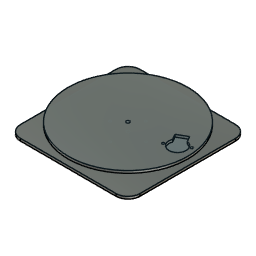
Bases v9 (Autodesk Fusion 360 design; units mm, degrees)
Autodesk Fusion 360 part; units mm, degrees
sketch "Sketch1" plane through (0, 0, 0) normal (0, 0, 1) x (1, 0, 0)
  line L0 (-100, 100) -> (100, 100)
  line L1 (100, 100) -> (100, -100)
  line L2 (100, -100) -> (-100, -100)
  line L3 (-100, -100) -> (-100, 100)
  circle A0 centre (0, 0) radius 65 construction
  circle A1 centre (30, 0) radius 2
  circle A2 centre (0, 30) radius 2
  circle A3 centre (-30, 0) radius 2
  circle A4 centre (0, -30) radius 2
  circle A5 centre (0, 0) radius 2.8
  point P0 (0, -100)
  point P1 (-100, 0)
  dimension "d1" = 200
  dimension "d2" = 200
  dimension "d3" = 130
  dimension "d10" = 30
  dimension "d11" = 30
  dimension "d12" = 30
  dimension "d13" = 30
  dimension "d14" = 4
  dimension "d15" = 4
  dimension "d16" = 4
  dimension "d17" = 4
  dimension "d18" = 5.6
  constraint horizontal L0
  constraint vertical L1
  constraint horizontal L2
  constraint vertical L3
  constraint midpoint L2 P0
  constraint midpoint L3 P1
  constraint vertical A0.centre P0
  constraint horizontal A0.centre P1
  constraint coincident A0.centre A5.centre
  constraint horizontal A0.centre A1.centre
  constraint vertical A0.centre A2.centre
  constraint horizontal A0.centre A3.centre
  constraint vertical A0.centre A4.centre
  measures "d1" distance of L0.start L2.end
  measures "d2" distance of L1.end L2.end
  measures "d3" diameter of A0
  measures "d10" distance of A0.centre A1.centre
  measures "d11" distance of A0.centre A2.centre
  measures "d12" distance of A0.centre A3.centre
  measures "d13" distance of A0.centre A4.centre
  measures "d14" diameter of A1
  measures "d15" diameter of A2
  measures "d16" diameter of A3
  measures "d17" diameter of A4
  measures "d18" diameter of A5
sketch "Sketch2" plane through (0, 0, 0) normal (0, 0, 1) x (1, 0, 0)
  circle A0 centre (0, 0) radius 100
  circle A1 centre (76, 6.9282) radius 14.3
  line L0 (60.8446, -1.8218) -> (91.1554, 15.6782) construction
  circle A2 centre (60.8446, -1.8218) radius 2
  circle A3 centre (91.1554, 15.6782) radius 2
  line L1 (76, 6.9282) -> (80, 0) construction
  line L2 (-49.7, 60.3) -> (49.7, 60.3) construction
  line L3 (49.7, 60.3) -> (49.7, -60.3) construction
  line L4 (49.7, -60.3) -> (-49.7, -60.3) construction
  line L5 (-49.7, -60.3) -> (-49.7, 60.3) construction
  line L6 (0, 0) -> (0, 9) construction
  line L7 (57.4058, 21.1344) -> (72.9942, 30.1344)
  line L8 (72.9942, 30.1344) -> (83.7942, 11.4282)
  line L9 (83.7942, 11.4282) -> (68.2058, 2.4282) construction
  line L10 (68.2058, 2.4282) -> (57.4058, 21.1344)
  circle A4 centre (0, 0) radius 2.8
  point P0 (80, 0)
  point P1 (76, 6.9282)
  point P2 (92.673, 16.9809)
  point P3 (98.1351, 19.2223)
  point P4 (0, 60.3)
  point P5 (-49.7, 0)
  point P6 (76, 6.9282)
  dimension "d19" = 200
  dimension "d20" = 80
  dimension "d21" = 28.6
  dimension "d22" = 8
  dimension "d23" = 35
  dimension "d24" = 4
  dimension "d25" = 4
  dimension "d27" = 99.4
  dimension "d28" = 120.6
  dimension "d29" = 60
  dimension "d30" = 18
  dimension "d31" = 21.6
  dimension "d32" = 5.6
  constraint coincident A0.centre L6.start
  constraint horizontal A0.centre P0
  constraint coincident P6 L0
  constraint midpoint L0 P1
  constraint coincident P1 A1.centre
  constraint coincident L0.start A2.centre
  constraint coincident L0.end A3.centre
  constraint coincident A3 P2
  constraint coincident A0 P3
  constraint coincident P6 P1
  constraint coincident P0 L1.end
  constraint perpendicular L0 L1
  constraint horizontal L2
  constraint vertical L3
  constraint horizontal L4
  constraint vertical L5
  constraint midpoint L2 P4
  constraint midpoint L5 P5
  constraint vertical A0.centre P4
  constraint horizontal A0.centre P5
  constraint vertical L6
  constraint parallel L0 L7
  constraint parallel L7 L9
  constraint parallel L8 L10
  constraint perpendicular L7 L8
  constraint midpoint L9 P6
  measures "d19" diameter of A0
  measures "d20" distance of A0.centre P0
  measures "d21" diameter of A1
  measures "d22" distance of P0 P6
  measures "d23" distance of L0.start L0.end
  measures "d24" diameter of A2
  measures "d25" diameter of A3
  measures "d27" distance of L2.start L2.end
  measures "d28" distance of L2.start L4.end
  measures "d29" angle of L0 L6
  measures "d30" distance of L7.start L7.end
  measures "d31" distance of L7.end L8.end
  measures "d32" diameter of A4
extrude "Extrude1" add sketch "Sketch1" along normal blind 4 makes body 1
extrude "Extrude2" add sketch "Sketch2" along normal blind 4 from surface at 14 separate body makes body 2
fillet "Fillet1" radius 20 4 edges at (100, -100, 2) (-100, -100, 2) (-100, 100, 2) (100, 100, 2) on bodies 1
sketch "Sketch3" plane through (0, 0, 18) normal (0, 0, 1) x (-1, 0, 0)
  circle A0 centre (0, 0) radius 100
  circle A1 centre (-60.8446, 1.8218) radius 2
  circle A2 centre (-91.1554, -15.6782) radius 2
  arc A3 (-62.6495, -12.052) -> (-78.2379, -21.052) centre (-76, -6.9282) ccw
  line L0 (-62.6495, -12.052) -> (-57.4058, -21.1344)
  line L1 (-57.4058, -21.1344) -> (-72.9942, -30.1344)
  line L2 (-72.9942, -30.1344) -> (-78.2379, -21.052)
  circle A4 centre (0, 0) radius 2.8
sketch "Sketch4" plane through (0, 0, 4) normal (0, 0, 1) x (-1, 0, 0)
  arc A0 (-100, -80) -> (-80, -100) centre (-80, -80) ccw
  line L0 (-80, -100) -> (80, -100)
  arc A1 (80, -100) -> (100, -80) centre (80, -80) ccw
  line L1 (100, -80) -> (100, 80)
  arc A2 (100, 80) -> (80, 100) centre (80, 80) ccw
  line L2 (80, 100) -> (-80, 100)
  arc A3 (-80, 100) -> (-100, 80) centre (-80, 80) ccw
  line L3 (-100, 80) -> (-100, -80)
  circle A4 centre (30, 0) radius 2
  circle A5 centre (-30, 0) radius 2
  circle A6 centre (0, -30) radius 2
  circle A7 centre (0, 0) radius 2.8
  circle A8 centre (0, 30) radius 2
equation "ScrewDiameter = 4 mm"
equation "ScrewDistance = 30 mm"
equation "BigGearDiameter = 130 mm"
equation "SmallGearDiameter = 30 mm"
equation "ShaftDiameter = 5 mm"
equation "Clearance = 0.3 mm"
equation "d10 = ScrewDistance"
equation "d11 = ScrewDistance"
equation "d12 = ScrewDistance"
equation "d13 = ScrewDistance"
equation "d14 = ScrewDiameter"
equation "d15 = ScrewDiameter"
equation "d16 = ScrewDiameter"
equation "d17 = ScrewDiameter"
equation "d18 = ShaftDiameter + Clearance * 2"
equation "d21 = 28 mm + 2 * Clearance"
equation "d24 = ScrewDiameter"
equation "d25 = ScrewDiameter"
equation "d30 = 17.4 mm + 2 * Clearance"
equation "d31 = 17 mm + Clearance + 4.3 mm"
equation "d32 = ShaftDiameter + 2 * Clearance"
